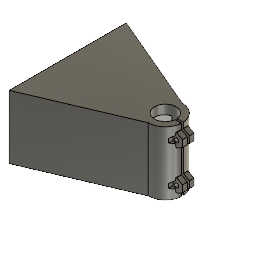
funnel (Autodesk Fusion 360 design; units mm, degrees)
Autodesk Fusion 360 part; units mm, degrees
sketch "Sketch1" plane through (0, 0, 0) normal (0, 0, 1) x (1, 0, 0)
  circle A0 centre (0, 0) radius 11
  circle A1 centre (0, 0) radius 17.5
  dimension "d1" = 22
  dimension "d2" = 35
  measures "d1" diameter of A0
  measures "d2" diameter of A1
extrude "Extrude1" add sketch "Sketch1" along normal blind 65 makes body 1
sketch "Sketch2" plane through (0, 0, 0) normal (0, 1, 0) x (1, 0, 0)
  line L0 (-17.5, 0) -> (17.5, 0)
  line L1 (0, 0) -> (17.491, 0)
  line L2 (-17.5, -65) -> (17.5, -65)
  line L3 (17.491, 0) -> (17.491, -65)
  line L4 (23.501, -9.0533) -> (17.5111, -5.5718)
  line L5 (17.5111, -5.5718) -> (11.501, -9.0185)
  line L6 (11.501, -9.0185) -> (11.481, -15.9467)
  line L7 (11.481, -15.9467) -> (17.4709, -19.4282)
  line L8 (17.4709, -19.4282) -> (23.4809, -15.9815)
  line L9 (23.4809, -15.9815) -> (23.501, -9.0533)
  line L10 (23.4967, -49.0458) -> (17.5025, -45.5718)
  line L11 (17.5025, -45.5718) -> (11.4967, -49.026)
  line L12 (11.4967, -49.026) -> (11.4852, -55.9542)
  line L13 (11.4852, -55.9542) -> (17.4795, -59.4282)
  line L14 (17.4795, -59.4282) -> (23.4852, -55.974)
  line L15 (23.4852, -55.974) -> (23.4967, -49.0458)
  point P0 (17.491, -12.5)
  point P1 (17.491, -52.5)
  dimension "d5" = 40
  dimension "d6" = 12.5
  measures "d5" distance of P0 P1
  measures "d6" distance of L0.end P0
extrude "Extrude2" add sketch "Sketch2" along normal mid plane 12 bodies 1
sketch "Sketch3" plane through (0, -6, 0) normal (0, -1, 0) x (1, 0, 0)
  line L0 (16.4393, 58.8253) -> (16.4393, 46.1833)
  line L1 (16.4393, 46.1833) -> (17.5025, 45.5718)
  line L2 (17.5025, 45.5718) -> (23.4967, 49.0458)
  line L3 (23.4967, 49.0458) -> (23.4852, 55.974)
  line L4 (23.4852, 55.974) -> (17.4795, 59.4282)
  line L5 (17.4795, 59.4282) -> (16.4393, 58.8253)
  line L6 (21.2573, 54.7808) -> (17.5573, 56.917)
  line L7 (17.5573, 56.917) -> (13.8573, 54.7808)
  line L8 (13.8573, 54.7808) -> (13.8573, 50.5084)
  line L9 (13.8573, 50.5084) -> (17.5573, 48.3723)
  line L10 (17.5573, 48.3723) -> (21.2573, 50.5084)
  line L11 (21.2573, 50.5084) -> (21.2573, 54.7808)
  line L12 (21.1909, 14.6516) -> (17.4909, 16.7878)
  line L13 (17.4909, 16.7878) -> (13.7909, 14.6516)
  line L14 (13.7909, 14.6516) -> (13.7909, 10.3792)
  line L15 (13.7909, 10.3792) -> (17.4909, 8.243)
  line L16 (17.4909, 8.243) -> (21.1909, 10.3792)
  line L17 (21.1909, 10.3792) -> (21.1909, 14.6516)
  line L18 (17.4709, 19.4282) -> (17.5111, 5.5718)
  line L19 (23.4809, 15.9815) -> (23.501, 9.0533)
  line L20 (23.491, 12.5174) -> (17.4909, 12.5154)
  point P0 (17.5573, 52.6446)
  point P1 (17.4909, 12.5154)
  point P2 (17.4709, 19.4282)
  point P3 (17.5111, 5.5718)
  dimension "d9" = 7.4
  dimension "d10" = 7.4
  measures "d9" distance of L6 L9
  measures "d10" distance of L14 L17
extrude "Extrude3" cut sketch "Sketch3" along normal blind 30 contours L0 L6 L7 L9 L10 L11 | L0 L7 L8 L9 | L12 L13 L17 L18 L20 | L16 L17 L18 L20 | L13 L14 L15 L16 L18 bodies 1
sketch "Sketch4" plane through (0, 6, 0) normal (0, 1, 0) x (-1, 0, 0)
  line L0 (-16.4393, 46.1833) -> (-16.4393, 58.8253)
  line L1 (-16.4393, 58.8253) -> (-17.4795, 59.4282)
  line L2 (-17.4795, 59.4282) -> (-23.4852, 55.974)
  line L3 (-23.4852, 55.974) -> (-23.4967, 49.0458)
  line L4 (-23.4967, 49.0458) -> (-17.5025, 45.5718)
  line L5 (-17.5025, 45.5718) -> (-16.4393, 46.1833)
  line L6 (-17.4795, 59.4282) -> (-17.5025, 45.5718)
  line L7 (-17.4709, 19.4282) -> (-17.5111, 5.5718)
  circle A0 centre (-17.491, 52.5) radius 4
  circle A1 centre (-17.491, 12.5) radius 4
  point P0 (-17.4709, 19.4282)
  point P1 (-17.5111, 5.5718)
  dimension "d13" = 8
  dimension "d14" = 8
  measures "d13" diameter of A0
  measures "d14" diameter of A1
extrude "Extrude4" cut sketch "Sketch4" along normal blind 15 contours L0 L6 A0 | L0 A0 | L6 A0 | L7 A1 | L7 A1 bodies 1
sketch "Sketch5" plane through (0, 6, 0) normal (0, 1, 0) x (-1, 0, 0)
  line L0 (-16.4393, 56.3593) -> (-16.4393, 58.8253)
  line L1 (-16.4393, 58.8253) -> (-17.4795, 59.4282)
  line L2 (-17.4795, 59.4282) -> (-23.4852, 55.974)
  line L3 (-23.4852, 55.974) -> (-23.4967, 49.0458)
  line L4 (-23.4967, 49.0458) -> (-17.5025, 45.5718)
  line L5 (-17.5025, 45.5718) -> (-16.4393, 46.1833)
  line L6 (-16.4393, 46.1833) -> (-16.4393, 48.6407)
  arc A0 (-16.4393, 48.6407) -> (-16.4393, 56.3593) centre (-17.491, 52.5) ccw
  circle A1 centre (-17.491, 52.5) radius 2.15
  circle A2 centre (-17.4709, 12.5) radius 2.15
  dimension "d17" = 4.3
  dimension "d18" = 4.3
  measures "d17" diameter of A1
  measures "d18" diameter of A2
extrude "Extrude5" cut sketch "Sketch5" against normal blind 15 contours A1 | A2 bodies 1
sketch "Sketch7" plane through (0, 0, 0) normal (1, 0, 0) x (0, 1, 0)
  line L0 (-1, 0) -> (1, 0)
  line L1 (1, 0) -> (1, 67.8352)
  line L2 (1, 67.8352) -> (-1, 67.8352)
  line L3 (-1, 67.8352) -> (-1, 0)
  line L4 (-11, 0) -> (11, 0)
  line L5 (17.5, 0) -> (-17.5, 0)
  dimension "d25" = 2
  dimension "d26" = 1
  measures "d25" distance of L1.end L2.end
  measures "d26" distance of L0.end origin
extrude "Extrude7" cut sketch "Sketch7" along normal blind 35 bodies 1
sketch "Sketch8" plane through (0, 0, 0) normal (1, 0, 0) x (0, 1, 0)
  line L0 (-8.5, 55) -> (8.5, 55)
  line L1 (8.5, 55) -> (8.5, 10)
  line L2 (8.5, 10) -> (-8.5, 10)
  line L3 (-8.5, 10) -> (-8.5, 55)
  line L4 (-8.5, 55) -> (8.5, 10) construction
  line L5 (8.5, 55) -> (-8.5, 10) construction
  line L6 (1, 45.5897) -> (1, 19.4279)
  line L7 (-17.5, 65) -> (17.5, 65)
  line L8 (17.5, 65) -> (17.5, 0)
  line L9 (17.5, 0) -> (-17.5, 0)
  line L10 (-17.5, 0) -> (-17.5, 65)
  line L11 (-17.5, 65) -> (17.5, 0) construction
  line L12 (17.5, 65) -> (-17.5, 0) construction
  point P0 (0, 32.5)
  point P1 (0, 32.5)
  point P2 (1, 0)
  dimension "d29" = 45
  dimension "d30" = 17
  dimension "d40" = 65
  dimension "d41" = 35
  dimension "d42" = 32.5
  measures "d29" distance of L0.end L1.end
  measures "d30" distance of L1.end L2.end
  measures "d40" distance of L7.start L9.end
  measures "d41" distance of L8.end L9.end
  measures "d42" distance of P1 P2
ref_plane "WorkPlane1" through (-100, 0, 0) normal (1, 0, 0) x (0, 1, 0)
sketch "Sketch9" plane through (-100, 0, 0) normal (1, 0, 0) x (0, 1, 0)
  line L0 (60, 0) -> (-60, 0)
  line L1 (-60, 0) -> (-60, 65)
  line L2 (-60, 65) -> (60, 65)
  line L3 (60, 65) -> (60, 0)
  line L4 (57, 3) -> (-57, 3)
  line L5 (-57, 3) -> (-57, 62)
  line L6 (-57, 62) -> (57, 62)
  line L7 (57, 62) -> (57, 3)
  dimension "d34" = 120
  dimension "d35" = 60
  dimension "d36" = 114
  dimension "d37" = 59
  dimension "d38" = 3
  dimension "d39" = 3
  dimension "d51" = 7
  dimension "d52" = 65
  measures "d34" distance of L0.start L0.end
  measures "d35" distance of origin L0.start
  measures "d36" distance of L4.start L4.end
  measures "d37" distance of L4.end L5.end
  measures "d38" distance of L2 L6
  measures "d39" distance of L1 L5
  measures "d52" distance of L0 L2
loft "Loft1" add profiles "Sketch9", "Sketch8" section 1 contours L0 L1 L2 L3 | L4 L5 L6 L7 section 2 contours L0 L1 L2 L3 | L7 L8 L9 L10 separate body makes body 2
loft "Loft2" cut profiles "Sketch8", "Sketch9" section 1 contours L0 L1 L2 L3 section 2 contours L4 L5 L6 L7 bodies 2 1
sketch "Sketch12" plane through (0, 0, 65) normal (0, 0, 1) x (-1, 0, 0)
  line L0 (100, -60) -> (100, 60)
  line L1 (100, 60) -> (0, 17.5)
  line L2 (0, 17.5) -> (0, -17.5)
  line L3 (0, -17.5) -> (100, -60)
  circle A0 centre (0, 0) radius 11
  arc A1 (-10.9545, -1) -> (-10.9545, 1) centre (0, 0) ccw
extrude "Extrude9" cut sketch "Sketch12" against normal blind 70 contours L2 A0 A1 | L2 A0 A1 bodies 2
combine "Combine1" operation add target body 2 tool bodies 1
sketch "Sketch14" plane through (-100, 0, 0) normal (-1, 0, 0) x (0, -1, 0)
  line L0 (60, 65) -> (-60, 65)
  line L1 (-60, 65) -> (-60, 0)
  line L2 (-60, 0) -> (60, 0)
  line L3 (60, 0) -> (60, 65)
  circle A0 centre (-67.1209, 72.0542) radius 14.4514
  circle A1 centre (-67.1209, -7.0542) radius 14.4514
  circle A2 centre (67.1209, -7.0542) radius 14.4514
  circle A3 centre (67.1209, 72.0542) radius 14.4514
  line L4 (57, 3) -> (-57, 3)
  line L5 (-57, 3) -> (-57, 62)
  line L6 (-57, 62) -> (57, 62)
  line L7 (57, 62) -> (57, 3)
extrude "Extrude11" [suppressed]
